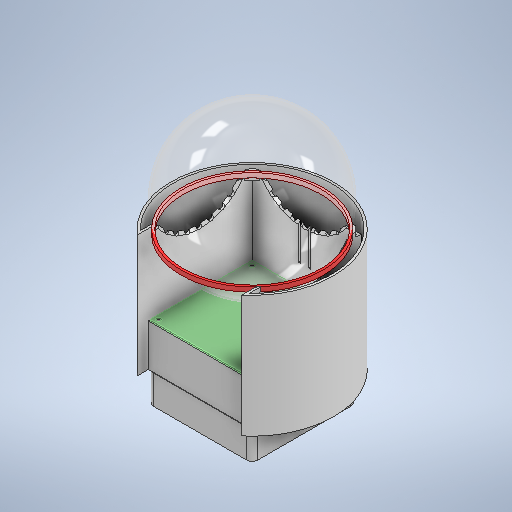
# Autodesk Inventor part: FanShroud
Saved by Autodesk Inventor 2025.2 (Build 292293000, 293)
## iProperties
Created: 2025-05-18
Part Number: FanShroud
Material: Generic
Document SubType Name: Modeling
Designer: user
Density: 1 g/cm^3
Appearance: Default
Author: user
## iProperties of the stored document FanShroud_3DPrint.ipt
Created: 2025-05-18
Part Number: FanShroud_3DPrint
Material: Generic
Document SubType Name: Modeling
Designer: user
Density: 1 g/cm^3
Appearance: Default
Author: user
Autodesk Inventor part; units mm, degrees
ref_plane "YZ Plane" through (0, 0, 0) normal (1, 0, 0) x (0, 1, 0)
ref_plane "XZ Plane" through (0, 0, 0) normal (0, 1, 0) x (-1, 0, 0)
ref_plane "XY Plane" through (0, 0, 0) normal (0, 0, 1) x (1, 0, 0)
sketch "Sketch1" plane through (0, 0, 0) normal (0, 1, 0) x (-1, 0, 0)
  line L0 (46, -46) -> (-46, -46)
  line L1 (-46, -46) -> (-46, 46)
  line L2 (-46, 46) -> (46, 46)
  line L3 (46, 46) -> (46, -46)
  line L4 (41.25, -41.25) -> (-41.25, -41.25) construction
  line L5 (-41.25, -41.25) -> (-41.25, 41.25) construction
  line L6 (-41.25, 41.25) -> (41.25, 41.25) construction
  line L7 (41.25, 41.25) -> (41.25, -41.25) construction
  circle A0 centre (41.25, -41.25) radius 2.25
  circle A1 centre (-41.25, -41.25) radius 2.25
  circle A2 centre (41.25, 41.25) radius 2.25
  circle A3 centre (-41.25, 41.25) radius 2.25
  circle A4 centre (0, 0) radius 44.5
  point P0 (0, -46)
  point P1 (-46, 0)
  point P2 (46, 0)
  point P3 (-41.25, 0)
  point P4 (0, -41.25)
  point P5 (41.25, 0)
  dimension "d1" = 92
  dimension "d2" = 82.5
  dimension "d3" = 4.5
  dimension "d4" = 4.5
  dimension "d5" = 4.5
  dimension "d6" = 4.5
  dimension "d7" = 89
  constraints: 16 end point, 6 midpoint, 5 centre point, 5 coincident, 4 parallel, 4 perpendicular, 2 horizontal, 2 horizontal alignment, 2 vertical alignment
  measures "d1" distance of point (-46, 0) point (46, 0)
  measures "d2" distance of point (-41.25, 0) point (41.25, 0)
  measures "d3" diameter of A0
  measures "d4" diameter of A1
  measures "d5" diameter of A2
  measures "d6" diameter of A3
  measures "d7" diameter of A4
extrude "Extrusion1" add sketch "Sketch1" along normal blind 25.4
fillet "Fillet1" radius 5 4 edges at (46, 12.7, 46) (46, 12.7, -46) (-46, 12.7, 46) (-46, 12.7, -46)
ref_plane "Work Plane1" through (0, 62.4, 0) normal (0, 1, 0) x (1, 0, 0)
sketch "Sketch2" plane through (0, 62.4, 0) normal (0, 1, 0) x (1, 0, 0)
  line L0 (45, 45) -> (-45, 45)
  line L1 (-45, 45) -> (-45, -45)
  line L2 (-45, -45) -> (45, -45)
  line L3 (45, -45) -> (45, 45)
  circle A0 centre (41.25, 41.25) radius 2.25 projected
  circle A1 centre (41.25, -41.25) radius 2.25 projected
  circle A2 centre (-41.25, -41.25) radius 2.25 projected
  circle A3 centre (-41.25, 41.25) radius 2.25 projected
  point P0 (0, 0)
  point P1 (0, 45)
  point P2 (45, 0)
  dimension "d12" = 90
  constraints: 8 end point, 2 midpoint, 2 parallel, 2 perpendicular, 1 horizontal, 1 horizontal alignment, 1 vertical alignment
  measures "d12" distance of L0.start L0.end
extrude "Extrusion2" add sketch "Sketch2" along normal blind 1.6 separate body
ref_plane "Work Plane2" through (0, 129, 0) normal (0, 1, 0) x (1, 0, 0)
sketch "Sketch4" plane through (0, 129, 0) normal (0, 1, 0) x (1, 0, 0)
  circle A0 centre (0, 0) radius 60.71
  circle A1 centre (0, 0) radius 62.71
  dimension "d16" = 121.42
  dimension "d17" = 2
  constraints: 2 centre point, 1 coincident
  measures "d16" diameter of A0
  measures "d17" radial gap between concentric circles of A0 A1
extrude "Extrusion3" add sketch "Sketch4" along normal blind 4 separate body
sketch "Sketch5" plane through (0, 0, 0) normal (0, 0, 1) x (1, 0, 0)
  circle A0 centre (0, 156.2227) radius 65
  line L0 (-41, 0) -> (41, 0) projected
  line L1 (-62.71, 129) -> (-62.71, 133) projected
  line L2 (-60.71, 133) -> (60.71, 133) projected
  line L3 (-60.71, 129) -> (60.71, 129) projected
  circle A1 centre (0, 156.2227) radius 63.5
  line L4 (0, 221.2227) -> (0, 91.2227)
  line L5 (0, -44.2445) -> (0, 265.4673) projected
  point P0 (0, 0)
  point P1 (0, 0)
  point P2 (0, 219.7227)
  point P3 (0, 92.7227)
  dimension "d20" = 130
  dimension "d21" = 1.5
  constraints: 3 point on circle, 2 centre point, 2 end point, 2 vertical alignment, 1 midpoint, 1 vertical
  measures "d20" diameter of A0
  measures "d21" radial gap between concentric circles of A0 A1
revolve "Revolution1" add sketch "Sketch5" angle 360 about axis through (0, -10, 0) along (0, 1, 0) separate body picked at (64.1708, 159.9851) picked at (58.1234, 129.44) picked at (54.4882, 122.9835) contours A0 L2 A1 L4 | A0 L3 A1 L2 | A0 L4 A1 L3
sketch "Sketch6" plane through (0, 64, 0) normal (0, 1, 0) x (1, 0, 0)
  line L0 (-45, 45) -> (-45, -45) projected
  line L1 (-45, -45) -> (45, -45) projected
  line L2 (45, -45) -> (45, 45) projected
  line L3 (45, 45) -> (-45, 45) projected
  circle A0 centre (41.25, 41.25) radius 2.25 projected
  circle A1 centre (41.25, -41.25) radius 2.25 projected
  circle A2 centre (-41.25, -41.25) radius 2.25 projected
  circle A3 centre (-41.25, 41.25) radius 2.25 projected
  line L4 (46, -46) -> (-46, -46)
  line L5 (-46, -46) -> (-46, 46)
  line L6 (-46, 46) -> (46, 46)
  line L7 (46, 46) -> (46, -46)
  line L8 (-48, 48) -> (-48, -48)
  line L9 (-48, -48) -> (48, -48)
  line L10 (48, -48) -> (48, 48)
  line L11 (48, 48) -> (-48, 48)
  circle A4 centre (0, 0) radius 65.0538
  circle A5 centre (0, 0) radius 67.8823
  line L12 (-46, -46) -> (-46, -48)
  line L13 (46, -46) -> (46, -48)
  dimension "d23" = 1
  dimension "d24" = 2
  constraints: 20 end point, 2 coincident, 2 perpendicular, 2 point on line, 12 other
  measures "d23" distance between parallel lines of L1 L4
  measures "d24" distance between parallel lines of L5 L8
extrude "Extrusion4" add sketch "Sketch6" along normal up to surface (65 mm away) separate body contours L7 A4 L10 | A4 L10 L9 L13 | A4 L8 L5 | L12 L9 L8 A4 | A4 L11 L10 | L6 A4 L11 | A4 L8 L11
sketch "Sketch7" plane through (0, 129, 0) normal (0, -1, 0) x (1, 0, 0)
  circle A0 centre (0, 0) radius 60.71 projected
  circle A1 centre (0, 0) radius 62.71 projected
  circle A2 centre (0, 0) radius 64.71
  line L0 (-48, 48) -> (-48, -48) projected
  line L1 (-48, -48) -> (-48, 48) projected
  line L2 (48, -48) -> (48, 48) projected
  line L3 (48, 48) -> (48, -48) projected
  line L4 (-46, 48) -> (-48, 48) projected
  line L5 (-46, -46) -> (-46, 48) projected
  line L6 (46, -46) -> (-46, -46) projected
  line L7 (46, 48) -> (46, -46) projected
  line L8 (48, 48) -> (46, 48) projected
  line L9 (48, -48) -> (48, 48) projected
  line L10 (-48, -48) -> (48, -48) projected
  line L11 (-48, 48) -> (-48, -48) projected
  point P0 (48, 43.398)
  point P1 (48, 37.1713)
  point P2 (-48, 37.1713)
  point P3 (-48, 43.398)
  point P4 (-48, 40.3552)
  point P5 (48, 40.3552)
  point P6 (46, 45.5125)
  point P7 (46, 42.6209)
  point P8 (-46, 42.6209)
  point P9 (-46, 45.5125)
  dimension "d27" = 2
  constraints: 1 centre point
  measures "d27" radial gap between concentric circles of A1 A2
extrude "Extrusion5" add sketch "Sketch7" along normal blind 2 contours A0 L2 A1 | L2 A1 L7 A0 | L2 A2 A1 | L7 A1 L6 A0 | L2 A2 L7 A1 | L6 A1 L10 A0 | L7 A2 L6 A1 | A0 L0 A1 | L5 A1 L0 A0 | A0 L6 A1 L5 | L10 A1 A0 | L6 A2 L10 A1 | A0 L10 A1 L6 | A1 L0 A2 | L5 A2 L0 A1 | A1 L6 A2 L5 | L10 A2 A1 | A1 L10 A2 L6 picked at (46.8936, -39.5966) picked at (46.8929, -42.6318) picked at (-46.8936, -39.5966) picked at (-46.8929, -42.6318) bodies 5
extrude "Extrusion6" add sketch "Sketch7" against normal up to surface (4 mm away) contours L2 A2 A1 | A1 L7 A2 L2 | L2 A2 L7 A1 | L7 A2 L6 A1 | A1 L0 A2 L5 | L6 A2 L10 A1 | A1 L0 A2 | L5 A2 L0 A1 | A1 L6 A2 L5 | L10 A2 A1 | A1 L10 A2 L6 bodies 5
sketch "Sketch8" plane through (0, 133, 0) normal (0, 1, 0) x (1, 0, 0)
  arc A0 (46, -45.5125) -> (-46, -45.5125) centre (0, 0) ccw projected
  circle A1 centre (0, 0) radius 69.71
  arc A2 (51.7089, -46.7512) -> (-51.7089, -46.7512) centre (0, 0) ccw construction
  circle A3 centre (0, 0) radius 71.71
  line L0 (-46, 39.6195) -> (-46, -48) projected
  line L1 (46, -48) -> (46, 39.6195) projected
  line L2 (-48, -48) -> (-48, -43.398) projected
  line L3 (-46, -48) -> (-48, -48) projected
  line L4 (-46, 39.6195) -> (-46, -42.6209) projected
  arc A4 (-39.6195, 46) -> (-46, 39.6195) centre (0, 0) ccw projected
  line L5 (39.6195, 46) -> (-39.6195, 46) projected
  arc A5 (46, 39.6195) -> (39.6195, 46) centre (0, 0) ccw projected
  line L6 (46, -48) -> (46, -45.5125) projected
  line L7 (48, -48) -> (46, -48) projected
  line L8 (48, -43.398) -> (48, -48) projected
  arc A6 (46, -42.6209) -> (-46, -42.6209) centre (0, 0) ccw projected
  line L9 (48, 37.1713) -> (48, -37.1713) projected
  arc A7 (48, -37.1713) -> (48, 37.1713) centre (0, 0) ccw projected
  line L10 (-37.1713, 48) -> (37.1713, 48) projected
  arc A8 (37.1713, 48) -> (-37.1713, 48) centre (0, 0) ccw projected
  arc A9 (-48, 37.1713) -> (-48, -37.1713) centre (0, 0) ccw projected
  line L11 (-48, -37.1713) -> (-48, 37.1713) projected
  arc A10 (-48, -43.398) -> (-46, -45.5125) centre (0, 0) ccw projected
  line L12 (-46, -45.5125) -> (-46, -48) projected
  line L13 (46, -42.6209) -> (46, 39.6195) projected
  arc A11 (46, -45.5125) -> (48, -43.398) centre (0, 0) ccw projected
  line L14 (-48, -48) -> (-46, -48)
  line L15 (-46, -48) -> (-46, -55.012)
  line L16 (-46, -55.012) -> (-48, -55.012)
  line L17 (-48, -55.012) -> (-48, -48)
  line L18 (46, -48) -> (48, -48)
  line L19 (48, -48) -> (48, -55.012)
  line L20 (48, -55.012) -> (46, -55.012)
  line L21 (46, -55.012) -> (46, -48)
  point P0 (-48, -43.398)
  point P1 (48, -43.398)
  point P2 (-46, -45.5125)
  point P3 (-48, -50.5518)
  point P4 (48, -50.5518)
  dimension "d32" = 5
  dimension "d33" = 2
  constraints: 16 end point, 4 parallel, 4 point on circle, 3 centre point, 2 collinear, 2 horizontal, 2 perpendicular, 1 coincident, 1 concentric
  measures "d32" radial gap between concentric circles of A0 A2
  measures "d33" radial gap between concentric circles of A1 A3
extrude "Extrusion7" add sketch "Sketch8" against normal up to surface (4 mm away) contours A0 L8 L7 L1 | A0 L0 L3 L2 bodies 5
extrude "Extrusion8" add sketch "Sketch8" against normal up to surface (69 mm away) contours L7 L19 A1 L21 | A1 L19 A3 L21 | L3 L15 A1 L17 | A1 L17 A3 L19 | L15 A3 L17 A1 bodies 5
sketch "Sketch9" plane through (0, 64, 0) normal (0, -1, 0) x (1, 0, 0)
  line L0 (-48, -48) -> (-48, 50.5518) projected
  line L1 (48, -48) -> (-48, -48) projected
  line L2 (48, -48) -> (48, 50.5518) projected
  arc A0 (-48, 50.5518) -> (48, 50.5518) centre (0, 0) ccw projected
  line L3 (-46, 55.012) -> (-46, -46) projected
  arc A1 (-46, 55.012) -> (46, 55.012) centre (0, 0) ccw projected
  line L4 (46, -46) -> (46, 55.012) projected
  line L5 (-46, -46) -> (46, -46) projected
extrude "Extrusion10" add sketch "Sketch9" along normal up to surface (1.6 mm away) bodies 5
sketch "Sketch11" plane through (0, 62.4, 0) normal (0, -1, 0) x (1, 0, 0)
  line L0 (-48, 45.5) -> (48, 45.5)
  line L1 (48, 45.5) -> (48, 43.5)
  line L2 (48, 43.5) -> (-48, 43.5)
  line L3 (-48, 43.5) -> (-48, 45.5)
  line L4 (-48, 50.5518) -> (-48, -48) projected
  line L5 (48, -48) -> (48, 50.5518) projected
  circle A0 centre (-41.25, 41.25) radius 2.25 projected
  line L6 (-48, -48) -> (48, -48) projected
  line L7 (48, -48) -> (48, 50.5518) projected
  arc A1 (-48, 50.5518) -> (48, 50.5518) centre (0, 0) ccw projected
  line L8 (-48, 50.5518) -> (-48, -48) projected
  arc A2 (-46, 55.012) -> (46, 55.012) centre (0, 0) ccw projected
  line L9 (46, 55.012) -> (46, -46) projected
  line L10 (46, -46) -> (-46, -46) projected
  line L11 (-46, -46) -> (-46, 55.012) projected
  point P0 (48, 50.5518)
  point P1 (-48, 50.5518)
  point P2 (-46, 45.5)
  point P3 (46, 45.5)
  point P4 (-48, -48)
  point P5 (48, -48)
  point P6 (48, 45.4993)
  point P7 (-48, 45.4991)
  dimension "d42" = 2
  constraints: 8 end point, 2 parallel, 2 point on line, 1 horizontal, 1 perpendicular, 1 tangent
  measures "d42" distance between parallel lines of L0 L2
extrude "Extrusion11" add sketch "Sketch11" along normal up to surface (37 mm away) contours L4 A1 L5 L0 L9 A2 L11 bodies 5
sketch "Sketch12" plane through (0, 25.4, 0) normal (0, 1, 0) x (1, 0, 0)
  arc A0 (-41, 46) -> (-46, 41) centre (-41, 41) ccw projected
  line L0 (-46, 41) -> (-46, -41) projected
  arc A1 (-46, -41) -> (-41, -46) centre (-41, -41) ccw projected
  line L1 (-41, -46) -> (41, -46) projected
  arc A2 (41, -46) -> (46, -41) centre (41, -41) ccw projected
  line L2 (46, -41) -> (46, 41) projected
  arc A3 (46, 41) -> (41, 46) centre (41, 41) ccw projected
  line L3 (41, 46) -> (-41, 46) projected
  circle A4 centre (0, 0) radius 44.5 projected
  circle A5 centre (41.25, -41.25) radius 2.25 projected
  circle A6 centre (-41.25, -41.25) radius 2.25 projected
  circle A7 centre (41.25, 41.25) radius 2.25 projected
  circle A8 centre (-41.25, 41.25) radius 2.25 projected
  circle A9 centre (0, 0) radius 71.71
  arc A10 (46, -55.012) -> (-46, -55.012) centre (0, 0) ccw projected
  circle A11 centre (-41.25, -41.25) radius 1.9
  circle A12 centre (-41.25, 41.25) radius 1.9
  circle A13 centre (41.25, 41.25) radius 1.9
  circle A14 centre (41.25, -41.25) radius 1.9
  circle A15 centre (-41.25, -41.25) radius 3.9
  circle A16 centre (-41.25, 41.25) radius 3.9
  circle A17 centre (41.25, -41.25) radius 3.9
  circle A18 centre (41.25, 41.25) radius 3.9
  dimension "d45" = 3.8
  dimension "d46" = 2
  dimension "d47" = 2
  dimension "d48" = 2
  dimension "d49" = 2
  constraints: 9 centre point, 5 coincident, 3 equal radius, 1 concentric
  measures "d45" diameter of A11
  measures "d46" radial gap between concentric circles of A11 A15
  measures "d47" radial gap between concentric circles of A12 A16
  measures "d48" radial gap between concentric circles of A14 A17
  measures "d49" radial gap between concentric circles of A13 A18
extrude "Extrusion12" add sketch "Sketch12" along normal up to surface (37 mm away) contours A5 | A6 | A7 | A8 | A15 | A16 | A17 | A18 bodies 5
extrude "Extrusion13" add sketch "Sketch12" along normal blind 3 contours L3 A3 L2 A2 L1 A1 L0 A0 | A9 bodies 5
extrude "Extrusion15" add sketch "Sketch11" along normal up to surface (34 mm away) contours L0 L11 L2 L3 | L2 L11 L10 L9 L5 L6 L4 | L0 L1 L2 L9 bodies 5
sketch "Sketch13" plane through (-46, 127, -39.6195) normal (1, 0, 0) x (0, 0, -1)
  circle A0 centre (-39.6195, -81.6) radius 10
  line L0 (-94.6315, 6) -> (-94.6315, -98.6) projected
  line L1 (6.3805, -64.6) -> (-94.6315, -64.6) projected
  line L2 (-94.6315, -98.6) -> (6.3805, -98.6) projected
  line L3 (-94.6315, -98.6) -> (-94.6315, -98.6) projected
  line L4 (6.3805, -98.6) -> (-94.6315, -98.6) projected
  line L5 (-84.1195, -98.6) -> (4.8805, -98.6) projected
  line L6 (-94.6315, -64.6) -> (-94.6315, -98.6) construction
  line L7 (-84.1195, -98.6) -> (4.8805, -98.6) construction
  line L8 (-84.1195, -101.6) -> (4.8805, -101.6) construction
  circle A1 centre (-14.6195, -81.6) radius 10
  circle A2 centre (-64.6195, -81.6) radius 10
  point P0 (-39.6195, -127)
  point P1 (-84.7695, -88.6)
  point P2 (-76.9695, -88.6)
  point P3 (-2.2695, -88.6)
  point P4 (5.5305, -88.6)
  point P5 (-84.7695, -88.6)
  point P6 (-76.9695, -88.6)
  point P7 (-2.2695, -88.6)
  point P8 (5.5305, -88.6)
  point P9 (-94.6315, -81.6)
  dimension "d58" = 20
  dimension "d59" = 20
  dimension "d60" = 20
  dimension "d61" = 25
  dimension "d62" = 25
  constraints: 3 centre point, 3 horizontal alignment, 2 end point, 1 midpoint, 1 perpendicular, 1 vertical alignment, 1 other
  measures "d58" diameter of A0
  measures "d59" diameter of A1
  measures "d60" diameter of A2
  measures "d61" distance of A2.centre A0.centre
  measures "d62" distance of A1.centre A0.centre
extrude "Extrusion16" cut sketch "Sketch13" against normal blind 3 bodies 5
pattern_circular "Circular Pattern1" count 3 over 180 about axis through (0, -10, 0) along (0, -1, 0) of "Extrusion16" bodies 5
extrude "Extrusion17" add sketch "Sketch11" along normal up to surface (34 mm away) contours L0 L11 L2 L3 | L0 L9 L2 L11 | L0 L1 L2 L9 bodies 5
revolve "Revolution2" cut sketch "Sketch5" angle 360 about axis through (0, -10, 0) along (0, 1, 0) picked at (-52.6944, 192.2524) picked at (-58.1234, 129.44) picked at (-3.7235, 190.485) picked at (-54.4882, 122.9835) picked at (-19.1229, 130.3333) picked at (-36.5426, 126.05) bodies 5 contours L4 A1 L2 A0 | L2 A1 L3 A0 | L4 L2 A1 | L3 A1 L4 A0 | L2 L4 L3 A1 | L3 L4 A1
sketch "Sketch14" plane through (0, 127, 0) normal (0, -1, 0) x (1, 0, 0)
  line L0 (37.1713, -48) -> (43.398, -48) projected
  arc A0 (-37.1713, -48) -> (37.1713, -48) centre (0, 0) ccw projected
  line L1 (-43.398, -48) -> (-37.1713, -48) projected
  arc A1 (-43.398, -48) -> (43.398, -48) centre (0, 0) ccw projected
  line L2 (-48, -37.1713) -> (-48, -43.398) projected
  arc A2 (-48, 37.1713) -> (-48, -37.1713) centre (0, 0) ccw projected
  line L3 (-48, 43.398) -> (-48, 37.1713) projected
  arc A3 (-48, 43.398) -> (-48, -43.398) centre (0, 0) ccw projected
  line L4 (48, -43.398) -> (48, -37.1713) projected
  arc A4 (48, -43.398) -> (48, 43.398) centre (0, 0) ccw projected
  line L5 (48, 37.1713) -> (48, 43.398) projected
  arc A5 (48, -37.1713) -> (48, 37.1713) centre (0, 0) ccw projected
extrude "Extrusion18" cut sketch "Sketch14" against normal blind 10 bodies 5
sketch "Sketch15" plane through (0, 28.4, 0) normal (0, 1, 0) x (1, 0, 0)
  line L0 (46, -45.5) -> (-46, -45.5) projected
  line L1 (-46, -55.012) -> (-46, -45.5) projected
  arc A0 (-46, -55.012) -> (46, -55.012) centre (0, 0) ccw projected
  line L2 (46, -45.5) -> (46, -55.012) projected
extrude "Extrusion19" cut sketch "Sketch15" against normal up to surface (3 mm away) bodies 5
sketch "Sketch18" plane through (-45.5125, 127, -46) normal (0, 0, 1) x (1, 0, 0)
  arc A0 (11.1625, 2) -> (79.8625, 2) centre (45.5125, 29.2227) ccw projected
  circle A1 centre (45.5125, -14.6065) radius 2.5
  circle A2 centre (55.6202, -13.425) radius 2.5
  circle A3 centre (35.4047, -13.425) radius 2.5
  circle A4 centre (65.183, -9.9445) radius 2.5
  circle A5 centre (25.8419, -9.9445) radius 2.5
  circle A6 centre (73.6853, -4.3524) radius 2.5
  circle A7 centre (17.3396, -4.3524) radius 2.5
  point P0 (45.5125, -127)
  dimension "d81" = 5
  dimension "d84" = 80
  constraints: 7 centre point, 1 point on circle, 13 other
  measures "d81" diameter of A1
extrude "Extrusion20" cut sketch "Sketch18" against normal up to surface (2 mm away) bodies 5
pattern_circular "Circular Pattern2" count 3 over 180 about axis through (0, -10, 0) along (0, 1, 0) of "Extrusion20" both ways yes bodies 5
sketch "Sketch17" plane through (-45.5125, 127, -46) normal (0, 0, 1) x (1, 0, 0)
  line L0 (42.0125, 2) -> (49.0125, 2)
  line L1 (49.0125, 2) -> (49.0125, -63)
  line L2 (49.0125, -63) -> (42.0125, -63)
  line L3 (42.0125, -63) -> (42.0125, 2)
  line L4 (91.5125, -64.6) -> (-0.4875, -64.6) projected
  line L5 (40.0125, 2) -> (51.0125, 2)
  line L6 (51.0125, 2) -> (51.0125, -63)
  line L7 (51.0125, -63) -> (40.0125, -63)
  line L8 (40.0125, -63) -> (40.0125, 2)
  line L9 (40.0125, -45) -> (51.0125, -45)
  line L10 (90.5125, -63) -> (0.5125, -63) projected
  point P0 (45.5125, -127)
  point P1 (45.5125, -63)
  point P2 (45.5125, -64.6)
  point P3 (45.5125, -63)
  point P4 (49.0125, -45)
  point P5 (42.0125, -45)
  dimension "d75" = 7
  dimension "d76" = 11
  dimension "d77" = 18
  dimension "d78" = 65
  constraints: 18 end point, 4 parallel, 3 collinear, 3 midpoint, 3 perpendicular, 2 horizontal, 2 point on line, 1 coincident, 1 vertical alignment
  measures "d75" distance of L0.start L0.end
  measures "d76" distance of L5.start L5.end
  measures "d77" distance between parallel lines of L9 L2
  measures "d78" distance between parallel lines of L0 L2
extrude "Extrusion21" cut sketch "Sketch17" against normal up to surface (2 mm away) contours L3 L9 L8 L5 | L5 L6 L9 L1 bodies 5
equation "\"d16\" = 130 * dRatio"
equation "\"d20\" = dGlobe"
equation "\"d45\" = dScrewHole"
equation "\"dRatio\" = 0.934"
equation "\"dGlobe\" = 130"
equation "\"dScrewHole\" = 3.8"
